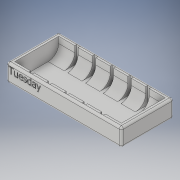
# Autodesk Inventor part: Tuesday
Saved by Autodesk Inventor 2019.4 (Build 234330000, 330)
## iProperties
Created: 2020-10-20
Part Number: Tuesday
Material: Generic
Document SubType Name: Modeling
Designer: daanswinters
Density: 1 g/cm^3
Appearance: Default
Author: daanswinters
Autodesk Inventor part; units mm, degrees
ref_plane "YZ Plane" through (0, 0, 0) normal (1, 0, 0) x (0, 1, 0)
ref_plane "XZ Plane" through (0, 0, 0) normal (0, 1, 0) x (-1, 0, 0)
ref_plane "XY Plane" through (0, 0, 0) normal (0, 0, 1) x (1, 0, 0)
sketch "Sketch1" plane through (0, 0, 0) normal (0, 0, 1) x (1, 0, 0)
  line L0 (55, -8.5) -> (-55, -8.5)
  line L1 (-55, -8.5) -> (-55, 8.5)
  line L2 (-55, 8.5) -> (55, 8.5)
  line L3 (55, 8.5) -> (55, -8.5)
  line L4 (55, -8.5) -> (-55, 8.5) construction
  line L5 (-55, -8.5) -> (55, 8.5) construction
  point P0 (0, 0)
  dimension "d0" = 110
  dimension "d1" = 17
  constraints: 12 end point, 2 midpoint, 2 parallel, 1 horizontal, 1 perpendicular
  measures "d0" distance of L1.end L2.end
  measures "d1" distance of L0.end L1.end
extrude "Extrusion1" add sketch "Sketch1" along normal blind 50
sketch "Sketch2" plane through (-55, 8.5, 0) normal (0, 1, 0) x (1, 0, 0)
  line L0 (0, 0) -> (0, -50) projected
  line L1 (110, -50) -> (0, -50)
  line L2 (0, -50) -> (0, 0)
  line L3 (0, 0) -> (110, 0)
  line L4 (110, 0) -> (110, -50)
  line L5 (110, -50) -> (0, 0) construction
  line L6 (0, -50) -> (110, 0) construction
  line L7 (106, -46) -> (106, -4)
  line L8 (4, -4) -> (4, -46)
  line L9 (56.15, -2) -> (53.85, -2)
  line L10 (53.85, -48) -> (56.15, -48)
  line L11 (56.15, -2) -> (53.85, -48) construction
  line L12 (53.85, -2) -> (56.15, -48) construction
  line L13 (73.15, -2) -> (70.85, -2)
  line L14 (70.85, -48) -> (73.15, -48)
  line L15 (73.15, -2) -> (70.85, -48) construction
  line L16 (70.85, -2) -> (73.15, -48) construction
  line L17 (0, -25) -> (110, -25) construction
  line L18 (87.85, -2) -> (90.15, -2)
  line L19 (90.15, -48) -> (87.85, -48)
  line L20 (87.85, -2) -> (90.15, -48) construction
  line L21 (90.15, -2) -> (87.85, -48) construction
  line L22 (36.85, -2) -> (39.15, -2)
  line L23 (39.15, -48) -> (36.85, -48)
  line L24 (36.85, -2) -> (39.15, -48) construction
  line L25 (39.15, -2) -> (36.85, -48) construction
  line L26 (19.85, -2) -> (22.15, -2)
  line L27 (22.15, -48) -> (19.85, -48)
  line L28 (19.85, -2) -> (22.15, -48) construction
  line L29 (22.15, -2) -> (19.85, -48) construction
  line L30 (90.15, -2) -> (90.15, -4)
  line L31 (90.15, -46) -> (90.15, -48)
  line L32 (87.85, -48) -> (87.85, -46)
  line L33 (87.85, -4) -> (87.85, -2)
  line L34 (73.15, -48) -> (73.15, -46)
  line L35 (73.15, -4) -> (73.15, -2)
  line L36 (70.85, -2) -> (70.85, -4)
  line L37 (70.85, -46) -> (70.85, -48)
  line L38 (56.15, -4) -> (56.15, -2)
  line L39 (53.85, -2) -> (53.85, -4)
  line L40 (53.85, -46) -> (53.85, -48)
  line L41 (56.15, -48) -> (56.15, -46)
  line L42 (39.15, -2) -> (39.15, -4)
  line L43 (39.15, -46) -> (39.15, -48)
  line L44 (36.85, -48) -> (36.85, -46)
  line L45 (36.85, -4) -> (36.85, -2)
  line L46 (22.15, -2) -> (22.15, -4)
  line L47 (19.85, -48) -> (19.85, -46)
  line L48 (19.85, -4) -> (19.85, -2)
  line L49 (22.15, -46) -> (22.15, -48)
  line L50 (4, -46) -> (19.95, -46)
  line L51 (22.05, -46) -> (36.95, -46)
  line L52 (39.05, -46) -> (53.95, -46)
  line L53 (56.05, -46) -> (70.95, -46)
  line L54 (73.05, -46) -> (87.95, -46)
  line L55 (90.05, -46) -> (106, -46)
  line L56 (106, -4) -> (90.05, -4)
  line L57 (87.95, -4) -> (73.05, -4)
  line L58 (70.95, -4) -> (56.05, -4)
  line L59 (53.95, -4) -> (39.05, -4)
  line L60 (36.95, -4) -> (22.05, -4)
  line L61 (19.95, -4) -> (4, -4)
  point P0 (55, 0)
  point P1 (55, -25)
  point P2 (72, -25)
  point P3 (89, -25)
  point P4 (38, -25)
  point P5 (21, -25)
  dimension "d4" = 65.556
  dimension "d5" = 110
  dimension "d7" = 2.3
  dimension "d8" = 46
  dimension "d9" = 2.3
  dimension "d10" = 46
  dimension "d11" = 0
  dimension "d12" = 2.3
  dimension "d13" = 46
  dimension "d14" = 2.3
  dimension "d15" = 46
  dimension "d16" = 2.3
  dimension "d17" = 46
  dimension "d18" = 17
  dimension "d19" = 17
  dimension "d20" = 17
  dimension "d21" = 17
  dimension "d22" = 2.862
  dimension "d23" = 2.862
  dimension "d24" = 106
  dimension "d25" = 4
  dimension "d26" = 42
  dimension "d27" = 2
  dimension "d28" = 0
  dimension "d29" = 42
  dimension "d30" = 0
  dimension "d31" = 42
  dimension "d32" = 0
  dimension "d33" = 42
  dimension "d34" = 0
  dimension "d35" = 42
  dimension "d36" = 0
  dimension "d37" = 42
  constraints: 122 end point, 73 parallel, 43 point on line, 17 perpendicular, 14 midpoint, 6 horizontal
  measures "d4" angle of L5 L0
  measures "d5" distance between parallel lines of L4 L0
  measures "d7" distance of L10.end L10.start
  measures "d8" distance of L10.start L9.end
  measures "d9" distance of L14.end L14.start
  measures "d10" distance of L14.start L13.end
  measures "d11" distance from line of L17 point (72, -25)
  measures "d12" distance of L19.start L19.end
  measures "d13" distance of L18.end L19.start
  measures "d14" distance of L23.start L23.end
  measures "d15" distance of L22.end L23.start
  measures "d16" distance of L27.start L27.end
  measures "d17" distance of L26.end L27.start
  measures "d18" distance of point (72, -25) point (55, -25)
  measures "d19" distance of point (89, -25) point (72, -25)
  measures "d20" distance of point (38, -25) point (55, -25)
  measures "d21" distance of point (21, -25) point (38, -25)
  measures "d22" angle of L0 L20
  measures "d23" angle of L0 L21
  measures "d24" distance between parallel lines of L7 L0
  measures "d25" distance between parallel lines of L8 L0
  measures "d26" distance between parallel lines of L56 L55
  measures "d27" distance between parallel lines of L56 L18
  measures "d28" distance between parallel lines of L56 L57
  measures "d29" distance between parallel lines of L56 L54
  measures "d30" distance between parallel lines of L56 L58
  measures "d31" distance between parallel lines of L56 L53
  measures "d32" distance between parallel lines of L56 L59
  measures "d33" distance between parallel lines of L56 L52
  measures "d34" distance between parallel lines of L56 L60
  measures "d35" distance between parallel lines of L56 L51
  measures "d36" distance between parallel lines of L56 L61
  measures "d37" distance between parallel lines of L56 L50
extrude "Extrusion2" cut sketch "Sketch2" against normal blind 16 contours L55 L31 L19 L32 L54 L34 L14 L37 L53 L41 L10 L40 L52 L43 L23 L44 L51 L49 L27 L47 L50 L8 L61 L48 L26 L46 L60 L45 L22 L42 L59 L39 L9 L38 L58 L36 L13 L35 L57 L33 L18 L30 L56 L7
fillet "Fillet1" radius 2 12 edges at (-55, 0, 50) (-55, 0, 0) (55, 0, 50) (55, 0, 0) (0, 8.5, 50) (-55, 8.5, 25) (0, 8.5, 0) (55, 8.5, 25) (55, -8.5, 25) (0, -8.5, 50) (-55, -8.5, 25) (0, -8.5, 0)
fillet "Fillet2" radius 10 6 edges at (-43.075, -7.5, 4) (-25.5, -7.5, 4) (-8.5, -7.5, 4) (8.5, -7.5, 4) (25.5, -7.5, 4) (43.075, -7.5, 4)
sketch "Sketch3" plane through (35.15, 8.5, 4) normal (0, 1, 0) x (1, 0, 0)
  line L0 (-70.3, -44) -> (-70.3, -42) projected
  line L1 (-51, 2) -> (-53.3, 2)
  line L2 (-34, 2) -> (-34, 0) projected
  line L3 (-36.3, -44) -> (-36.3, -42) projected
  line L4 (-19.3, -44) -> (-19.3, -42) projected
  line L5 (-2.3, -44) -> (-2.3, -42) projected
  line L6 (0, 2) -> (0, 0) projected
  line L7 (-19.8, 2) -> (-16.5, 2)
  line L8 (-16.5, 2) -> (-16.5, -44)
  line L9 (-16.5, -44) -> (-19.8, -44)
  line L10 (-19.8, -44) -> (-19.8, 2)
  line L11 (-19.8, 2) -> (-16.5, -44) construction
  line L12 (-16.5, 2) -> (-19.8, -44) construction
  line L13 (-2.8, -44) -> (0.5, -44)
  line L14 (0.5, -44) -> (0.5, 2)
  line L15 (0.5, 2) -> (-2.8, 2)
  line L16 (-2.8, 2) -> (-2.8, -44)
  line L17 (-2.8, -44) -> (0.5, 2) construction
  line L18 (0.5, -44) -> (-2.8, 2) construction
  line L19 (-36.8, -44) -> (-33.5, -44)
  line L20 (-33.5, -44) -> (-33.5, 2)
  line L21 (-33.5, 2) -> (-36.8, 2)
  line L22 (-36.8, 2) -> (-36.8, -44)
  line L23 (-36.8, -44) -> (-33.5, 2) construction
  line L24 (-33.5, -44) -> (-36.8, 2) construction
  line L25 (-51, 2) -> (-36.3, 2) projected
  line L26 (-53.8, -44) -> (-50.5, -44)
  line L27 (-50.5, -44) -> (-50.5, 2)
  line L28 (-50.5, 2) -> (-53.8, 2)
  line L29 (-53.8, 2) -> (-53.8, -44)
  line L30 (-53.8, -44) -> (-50.5, 2) construction
  line L31 (-50.5, -44) -> (-53.8, 2) construction
  line L32 (-53.3, -44) -> (-68, -44) projected
  line L33 (-70.8, 2) -> (-67.5, 2)
  line L34 (-67.5, 2) -> (-67.5, -44)
  line L35 (-67.5, -44) -> (-70.8, -44)
  line L36 (-70.8, -44) -> (-70.8, 2)
  line L37 (-70.8, 2) -> (-67.5, -44) construction
  line L38 (-67.5, 2) -> (-70.8, -44) construction
  point P0 (-35.15, 4)
  point P1 (-68, 2)
  point P2 (-17, 2)
  point P3 (-18.15, -21)
  point P4 (-1.15, -21)
  point P5 (-35.15, -21)
  point P6 (-52.15, -21)
  point P7 (-69.15, -21)
  dimension "d42" = 3.3
  dimension "d43" = 46
  dimension "d44" = 3.3
  dimension "d45" = 3.3
  dimension "d46" = 3.3
  dimension "d47" = 3.3
  dimension "d48" = 90
  dimension "d49" = 0.5
  dimension "d50" = 16.5
  dimension "d51" = 33.5
  dimension "d52" = 50.5
  dimension "d53" = 67.5
  dimension "d54" = 46
  dimension "d55" = 0
  dimension "d56" = 53.3
  constraints: 62 end point, 14 parallel, 10 midpoint, 5 horizontal, 5 perpendicular, 3 point on line
  measures "d42" distance of L8.end L9.end
  measures "d43" distance of L7.end L8.end
  measures "d44" distance of L15.end L14.end
  measures "d45" distance of L21.end L20.end
  measures "d46" distance of L28.end L27.end
  measures "d47" distance of L34.end L35.end
  measures "d48" angle of L6 L1
  measures "d49" distance between parallel lines of L6 L14
  measures "d50" distance between parallel lines of L6 L8
  measures "d51" distance between parallel lines of L6 L20
  measures "d52" distance between parallel lines of L6 L27
  measures "d53" distance between parallel lines of L6 L34
  measures "d54" distance between parallel lines of L25 L9
  measures "d55" distance between parallel lines of L15 L25
  measures "d56" distance from line of L1.end L6
extrude "Extrusion3" cut sketch "Sketch3" against normal blind 16
sketch "Sketch4" plane through (0, 0, 50) normal (0, 0, 1) x (1, 0, 0)
  line L0 (-52.9749, 6.5012) -> (53.0345, 6.5012) construction
  line L1 (53.0345, 6.5012) -> (53.0345, -6.5247) construction
  line L2 (53.0345, -6.5247) -> (-52.9749, -6.5247) construction
  line L3 (-52.9749, -6.5247) -> (-52.9749, 6.5012) construction
  line L4 (-50.9334, 0.1294) -> (-50.9334, 5.5077)
  line L5 (-50.9334, 5.5077) -> (-52.9799, 5.5077)
  line L6 (-52.9799, 5.5077) -> (-52.9799, 6.2294)
  line L7 (-52.9799, 6.2294) -> (-48.0761, 6.2294)
  line L8 (-48.0761, 6.2294) -> (-48.0761, 5.5077)
  line L9 (-48.0761, 5.5077) -> (-50.1227, 5.5077)
  line L10 (-50.1227, 5.5077) -> (-50.1227, 0.1294)
  line L11 (-50.1227, 0.1294) -> (-50.9334, 0.1294)
  line L12 (-43.9584, 0.1294) -> (-44.7295, 0.1294)
  line L13 (-44.7295, 0.1294) -> (-44.7295, 0.6336)
  spline S0 degree 2 poles (-44.7295, 0.6336) (-45.0855, 0.3222) (-45.7231, 0.0008) (-46.1186, 0.0008) knots 0 0 0 1 2 2 2
  spline S1 degree 2 poles (-46.1186, 0.0008) (-46.4152, 0.0008) (-46.9441, 0.1986) (-47.1369, 0.4111) knots 0 0 0 1 2 2 2
  spline S2 degree 2 poles (-47.1369, 0.4111) (-47.3347, 0.6237) (-47.5522, 1.2713) (-47.5522, 1.7359) knots 0 0 0 1 2 2 2
  line L14 (-47.5522, 1.7359) -> (-47.5522, 4.7068)
  line L15 (-47.5522, 4.7068) -> (-46.781, 4.7068)
  line L16 (-46.781, 4.7068) -> (-46.781, 2.0968)
  spline S3 degree 2 poles (-46.781, 2.0968) (-46.781, 1.731) (-46.7266, 1.2515) (-46.6327, 1.0735) knots 0 0 0 1 2 2 2
  spline S4 degree 2 poles (-46.6327, 1.0735) (-46.5388, 0.8956) (-46.2175, 0.7324) (-45.9159, 0.7324) knots 0 0 0 1 2 2 2
  spline S5 degree 2 poles (-45.9159, 0.7324) (-45.6342, 0.7324) (-44.9965, 1.0538) (-44.7295, 1.2861) knots 0 0 0 1 2 2 2
  line L17 (-44.7295, 1.2861) -> (-44.7295, 4.7068)
  line L18 (-44.7295, 4.7068) -> (-43.9584, 4.7068)
  line L19 (-43.9584, 4.7068) -> (-43.9584, 0.1294)
  spline S6 degree 2 poles (-40.854, 0.0256) (-41.9514, 0.0256) (-43.1576, 1.2564) (-43.1576, 2.3934) knots 0 0 0 1 2 2 2
  spline S7 degree 2 poles (-43.1576, 2.3934) (-43.1576, 3.5106) (-41.986, 4.8354) (-41.0419, 4.8354) knots 0 0 0 1 2 2 2
  spline S8 degree 2 poles (-41.0419, 4.8354) (-40.6167, 4.8354) (-39.9593, 4.5882) (-39.7171, 4.3262) knots 0 0 0 1 2 2 2
  spline S9 degree 2 poles (-39.7171, 4.3262) (-39.4699, 4.0642) (-39.2079, 3.3079) (-39.2079, 2.7592) knots 0 0 0 1 2 2 2
  line L20 (-39.2079, 2.7592) -> (-39.2079, 2.339)
  line L21 (-39.2079, 2.339) -> (-42.3765, 2.339)
  spline S10 degree 2 poles (-42.3765, 2.339) (-42.3765, 1.5431) (-41.5757, 0.6978) (-40.8639, 0.6978) knots 0 0 0 1 2 2 2
  spline S11 degree 2 poles (-40.8639, 0.6978) (-40.6118, 0.6978) (-40.1224, 0.8115) (-39.9247, 0.9005) knots 0 0 0 1 2 2 2
  spline S12 degree 2 poles (-39.9247, 0.9005) (-39.7171, 0.9994) (-39.4304, 1.1724) (-39.3364, 1.2515) knots 0 0 0 1 2 2 2
  line L22 (-39.3364, 1.2515) -> (-39.2919, 1.2515)
  line L23 (-39.2919, 1.2515) -> (-39.2919, 0.4111)
  spline S13 degree 2 poles (-39.2919, 0.4111) (-39.4254, 0.3568) (-39.8308, 0.1986) (-39.9889, 0.1541) knots 0 0 0 1 2 2 2
  spline S14 degree 2 poles (-39.9889, 0.1541) (-40.2114, 0.0898) (-40.5772, 0.0256) (-40.854, 0.0256) knots 0 0 0 1 2 2 2
  spline S15 degree 2 poles (-39.9593, 2.9273) (-39.9692, 3.2387) (-40.0977, 3.6935) (-40.2213, 3.8467) knots 0 0 0 1 2 2 2
  spline S16 degree 2 poles (-40.2213, 3.8467) (-40.3547, 4.0197) (-40.7749, 4.2026) (-41.0864, 4.2026) knots 0 0 0 1 2 2 2
  spline S17 degree 2 poles (-41.0864, 4.2026) (-41.3928, 4.2026) (-41.8229, 4.0197) (-42.0009, 3.8418) knots 0 0 0 1 2 2 2
  spline S18 degree 2 poles (-42.0009, 3.8418) (-42.1739, 3.6589) (-42.3518, 3.2189) (-42.3765, 2.9273) knots 0 0 0 1 2 2 2
  line L24 (-42.3765, 2.9273) -> (-39.9593, 2.9273)
  spline S19 degree 2 poles (-37.1911, 0.0206) (-37.6508, 0.0206) (-38.4466, 0.2678) (-38.7086, 0.4062) knots 0 0 0 1 2 2 2
  line L25 (-38.7086, 0.4062) -> (-38.7086, 1.2713)
  line L26 (-38.7086, 1.2713) -> (-38.6691, 1.2713)
  spline S20 degree 2 poles (-38.6691, 1.2713) (-38.5702, 1.1922) (-38.3033, 1.0043) (-38.0808, 0.9005) knots 0 0 0 1 2 2 2
  spline S21 degree 2 poles (-38.0808, 0.9005) (-37.8881, 0.8066) (-37.4135, 0.6682) (-37.1614, 0.6682) knots 0 0 0 1 2 2 2
  spline S22 degree 2 poles (-37.1614, 0.6682) (-36.9785, 0.6682) (-36.5583, 0.7522) (-36.4594, 0.8214) knots 0 0 0 1 2 2 2
  spline S23 degree 2 poles (-36.4594, 0.8214) (-36.3161, 0.9153) (-36.1876, 1.1279) (-36.1876, 1.3454) knots 0 0 0 1 2 2 2
  spline S24 degree 2 poles (-36.1876, 1.3454) (-36.1876, 1.6173) (-36.4842, 1.8991) (-36.8648, 1.993) knots 0 0 0 1 2 2 2
  spline S25 degree 2 poles (-36.8648, 1.993) (-37.0131, 2.0276) (-37.4876, 2.1265) (-37.6903, 2.1808) knots 0 0 0 1 2 2 2
  spline S26 degree 2 poles (-37.6903, 2.1808) (-38.2143, 2.3341) (-38.6889, 2.9668) (-38.6889, 3.4166) knots 0 0 0 1 2 2 2
  spline S27 degree 2 poles (-38.6889, 3.4166) (-38.6889, 4.0395) (-37.7546, 4.8156) (-36.9834, 4.8156) knots 0 0 0 1 2 2 2
  spline S28 degree 2 poles (-36.9834, 4.8156) (-36.6028, 4.8156) (-35.8317, 4.6277) (-35.5697, 4.4844) knots 0 0 0 1 2 2 2
  line L27 (-35.5697, 4.4844) -> (-35.5697, 3.6589)
  line L28 (-35.5697, 3.6589) -> (-35.6092, 3.6589)
  spline S29 degree 2 poles (-35.6092, 3.6589) (-35.9058, 3.8961) (-36.6275, 4.168) (-36.9983, 4.168) knots 0 0 0 1 2 2 2
  spline S30 degree 2 poles (-36.9983, 4.168) (-37.3789, 4.168) (-37.9029, 3.8467) (-37.9029, 3.5254) knots 0 0 0 1 2 2 2
  spline S31 degree 2 poles (-37.9029, 3.5254) (-37.9029, 3.2337) (-37.5915, 2.952) (-37.2454, 2.863) knots 0 0 0 1 2 2 2
  spline S32 degree 2 poles (-37.2454, 2.863) (-37.0774, 2.8185) (-36.6522, 2.7295) (-36.4199, 2.6752) knots 0 0 0 1 2 2 2
  spline S33 degree 2 poles (-36.4199, 2.6752) (-35.9157, 2.5466) (-35.4016, 1.9584) (-35.4016, 1.4492) knots 0 0 0 1 2 2 2
  spline S34 degree 2 poles (-35.4016, 1.4492) (-35.4016, 1.1526) (-35.6339, 0.6286) (-35.8613, 0.4359) knots 0 0 0 1 2 2 2
  spline S35 degree 2 poles (-35.8613, 0.4359) (-36.1035, 0.2332) (-36.7214, 0.0206) (-37.1911, 0.0206) knots 0 0 0 1 2 2 2
  line L29 (-31.1652, 0.1294) -> (-31.9364, 0.1294)
  line L30 (-31.9364, 0.1294) -> (-31.9364, 0.594)
  spline S36 degree 2 poles (-31.9364, 0.594) (-32.1143, 0.4457) (-32.3763, 0.248) (-32.5543, 0.164) knots 0 0 0 1 2 2 2
  spline S37 degree 2 poles (-32.5543, 0.164) (-32.7174, 0.0849) (-33.0684, 0.0008) (-33.3007, 0.0008) knots 0 0 0 1 2 2 2
  spline S38 degree 2 poles (-33.3007, 0.0008) (-33.6764, 0.0008) (-34.3091, 0.3123) (-34.5316, 0.6138) knots 0 0 0 1 2 2 2
  spline S39 degree 2 poles (-34.5316, 0.6138) (-34.754, 0.9153) (-35.0012, 1.8051) (-35.0012, 2.3835) knots 0 0 0 1 2 2 2
  spline S40 degree 2 poles (-35.0012, 2.3835) (-35.0012, 2.9866) (-34.6898, 3.8665) (-34.4179, 4.1977) knots 0 0 0 1 2 2 2
  spline S41 degree 2 poles (-34.4179, 4.1977) (-34.1658, 4.4943) (-33.4589, 4.8354) (-33.0684, 4.8354) knots 0 0 0 1 2 2 2
  spline S42 degree 2 poles (-33.0684, 4.8354) (-32.7273, 4.8354) (-32.2181, 4.6821) (-31.9364, 4.5239) knots 0 0 0 1 2 2 2
  line L31 (-31.9364, 4.5239) -> (-31.9364, 6.5012)
  line L32 (-31.9364, 6.5012) -> (-31.1652, 6.5012)
  line L33 (-31.1652, 6.5012) -> (-31.1652, 0.1294)
  line L34 (-31.9364, 1.2416) -> (-31.9364, 3.8863)
  spline S43 degree 2 poles (-31.9364, 3.8863) (-32.2231, 4.0247) (-32.6778, 4.1285) (-32.9398, 4.1285) knots 0 0 0 1 2 2 2
  spline S44 degree 2 poles (-32.9398, 4.1285) (-33.533, 4.1285) (-34.2053, 3.2387) (-34.2053, 2.3983) knots 0 0 0 1 2 2 2
  spline S45 degree 2 poles (-34.2053, 2.3983) (-34.2053, 1.5876) (-33.6912, 0.7324) (-33.1227, 0.7324) knots 0 0 0 1 2 2 2
  spline S46 degree 2 poles (-33.1227, 0.7324) (-32.8212, 0.7324) (-32.2082, 1.0093) (-31.9364, 1.2416) knots 0 0 0 1 2 2 2
  spline S47 degree 2 poles (-27.4973, 0.6138) (-27.5912, 0.5446) (-27.9076, 0.2974) (-28.0559, 0.2233) knots 0 0 0 1 2 2 2
  spline S48 degree 2 poles (-28.0559, 0.2233) (-28.2586, 0.1145) (-28.6392, 0.0008) (-28.9852, 0.0008) knots 0 0 0 1 2 2 2
  spline S49 degree 2 poles (-28.9852, 0.0008) (-29.267, 0.0008) (-29.7761, 0.2134) (-29.9689, 0.4062) knots 0 0 0 1 2 2 2
  spline S50 degree 2 poles (-29.9689, 0.4062) (-30.1518, 0.594) (-30.3743, 1.1477) (-30.3743, 1.4542) knots 0 0 0 1 2 2 2
  spline S51 degree 2 poles (-30.3743, 1.4542) (-30.3743, 1.9287) (-29.9739, 2.601) (-29.5389, 2.7938) knots 0 0 0 1 2 2 2
  spline S52 degree 2 poles (-29.5389, 2.7938) (-29.1533, 2.9718) (-28.1053, 3.1052) (-27.4973, 3.1398) knots 0 0 0 1 2 2 2
  line L35 (-27.4973, 3.1398) -> (-27.4973, 3.2881)
  spline S53 degree 2 poles (-27.4973, 3.2881) (-27.4973, 3.5551) (-27.6604, 3.8863) (-27.8087, 3.9802) knots 0 0 0 1 2 2 2
  spline S54 degree 2 poles (-27.8087, 3.9802) (-27.957, 4.0741) (-28.3821, 4.1334) (-28.6095, 4.1334) knots 0 0 0 1 2 2 2
  spline S55 degree 2 poles (-28.6095, 4.1334) (-28.8765, 4.1334) (-29.5982, 3.9752) (-29.959, 3.822) knots 0 0 0 1 2 2 2
  line L36 (-29.959, 3.822) -> (-30.0035, 3.822)
  line L37 (-30.0035, 3.822) -> (-30.0035, 4.608)
  spline S56 degree 2 poles (-30.0035, 4.608) (-29.791, 4.6673) (-28.9951, 4.8156) (-28.6046, 4.8156) knots 0 0 0 1 2 2 2
  spline S57 degree 2 poles (-28.6046, 4.8156) (-28.13, 4.8156) (-27.4825, 4.6673) (-27.2254, 4.4745) knots 0 0 0 1 2 2 2
  spline S58 degree 2 poles (-27.2254, 4.4745) (-26.9733, 4.2867) (-26.7261, 3.6885) (-26.7261, 3.2585) knots 0 0 0 1 2 2 2
  line L38 (-26.7261, 3.2585) -> (-26.7261, 0.1294)
  line L39 (-26.7261, 0.1294) -> (-27.4973, 0.1294)
  line L40 (-27.4973, 0.1294) -> (-27.4973, 0.6138)
  line L41 (-27.4973, 1.2564) -> (-27.4973, 2.5269)
  spline S59 degree 2 poles (-27.4973, 2.5269) (-27.7741, 2.5021) (-28.6095, 2.4181) (-28.8715, 2.339) knots 0 0 0 1 2 2 2
  spline S60 degree 2 poles (-28.8715, 2.339) (-29.178, 2.2451) (-29.5784, 1.8546) (-29.5784, 1.5085) knots 0 0 0 1 2 2 2
  spline S61 degree 2 poles (-29.5784, 1.5085) (-29.5784, 1.1131) (-29.1335, 0.7127) (-28.7084, 0.7127) knots 0 0 0 1 2 2 2
  spline S62 degree 2 poles (-28.7084, 0.7127) (-28.3475, 0.7127) (-27.7543, 1.0241) (-27.4973, 1.2564) knots 0 0 0 1 2 2 2
  line L42 (-22.0498, 4.7068) -> (-24.5116, -1.5563)
  line L43 (-24.5116, -1.5563) -> (-25.3371, -1.5563)
  line L44 (-25.3371, -1.5563) -> (-24.5165, 0.3518)
  line L45 (-24.5165, 0.3518) -> (-26.1774, 4.7068)
  line L46 (-26.1774, 4.7068) -> (-25.347, 4.7068)
  line L47 (-25.347, 4.7068) -> (-24.0963, 1.3158)
  line L48 (-24.0963, 1.3158) -> (-22.8506, 4.7068)
  line L49 (-22.8506, 4.7068) -> (-22.0498, 4.7068)
  point P0 (0, 0)
  constraints: 2 other
extrude "Extrusion4" cut sketch "Sketch4" against normal blind 0.5
fillet "Fillet3" radius 10 6 edges at (-43.325, -7.5, 46) (-25.5, -7.5, 46) (-8.5, -7.5, 46) (8.5, -7.5, 46) (25.5, -7.5, 46) (43.325, -7.5, 46)
body "Solid1"
